Autodesk Inventor part; units mm, degrees
(part 3 of 6)
  line L915 (89.0625, 287.8731) -> (89.2677, 288.1729) construction
  line L916 (89.2677, 288.1729) -> (89.7412, 288.6466) construction
  line L917 (89.7412, 288.6466) -> (90.0412, 288.8519) construction
  line L918 (90.0412, 288.8519) -> (90.6984, 289.1241) construction
  line L919 (90.6984, 289.1241) -> (91.0556, 289.191) construction
  line L920 (91.0556, 289.191) -> (91.7253, 289.191) construction
  line L921 (91.7253, 289.191) -> (92.0826, 289.1241) construction
  line L922 (92.0826, 289.1241) -> (92.7397, 288.8518) construction
  line L923 (92.7397, 288.8518) -> (93.0397, 288.6465) construction
  line L924 (93.0397, 288.6465) -> (93.5132, 288.1729) construction
  line L925 (93.5132, 288.1729) -> (93.7184, 287.8731) construction
  line L926 (93.7184, 287.8731) -> (93.9905, 287.216) construction
  line L927 (93.9905, 287.216) -> (94.0574, 286.8589) construction
  line L928 (94.0574, 286.8589) -> (94.0574, 286.524) construction
  arc A169 (91.0729, 293.509) -> (84.7229, 287.159) centre (91.0729, 287.159) ccw
  arc A170 (98.6893, 291.9215) -> (97.1018, 293.509) centre (97.1018, 291.9215) ccw
  line L929 (97.1018, 293.509) -> (91.0729, 293.509)
  arc A171 (56.7829, 285.836) -> (57.2679, 280.4634) centre (86.7829, 285.836) ccw
  arc A172 (57.7529, 275.0908) -> (57.2679, 280.4634) centre (27.7529, 275.0908) ccw
  circle A173 centre (54.7529, 269.1865) radius 1.25
  arc A174 (61.7529, 277.269) -> (59.7529, 277.269) centre (60.7529, 277.269) ccw
  point P0 (0, 0)
  constraints: 242 point on circle, 232 end point, 175 centre point, 64 other
extrude "Extrusion1" add sketch "Sketch1" along normal blind 3.175
sketch "Sketch4" plane through (0, 3.175, 0) normal (0, 1, 0) x (1, 0, 0)
  line L0 (68.0533, -173.3296) -> (67.2896, -175.455) construction
  line L1 (67.2896, -175.455) -> (65.953, -179.1748) construction
  line L2 (65.953, -179.1748) -> (66.2895, -184.0091) construction
  line L3 (66.2895, -184.0091) -> (66.4824, -187.911) construction
  line L4 (66.4824, -187.911) -> (66.5623, -189.5259) construction
  line L5 (66.5623, -189.5259) -> (66.4659, -191.8029) construction
  line L6 (66.4659, -191.8029) -> (67.3465, -193.2223) construction
  line L7 (67.3465, -193.2223) -> (68.1874, -194.5775) construction
  line L8 (68.1874, -194.5775) -> (69.7981, -195.2031) construction
  line L9 (69.7981, -195.2031) -> (71.183, -194.3094) construction
  line L10 (71.183, -194.3094) -> (72.3101, -193.582) construction
  spline S0 degree 3 poles (71.4379, -191.0403) (71.4136, -190.7511) (71.3322, -190.3365) (71.3219, -190.1438) knots 8.458233 8.458233 8.458233 8.458233 9 9 9 9
  line L11 (71.3322, -190.3365) -> (71.3219, -190.1438) construction
  spline S1 degree 3 poles (71.3219, -190.1438) (71.2889, -189.5237) (71.258, -188.9035) (71.2265, -188.2833) knots 9 9 9 9 10 10 10 10
  line L12 (71.3219, -190.1438) -> (71.2889, -189.5237) construction
  line L13 (71.2889, -189.5237) -> (71.258, -188.9035) construction
  line L14 (71.258, -188.9035) -> (71.2265, -188.2833) construction
  line L15 (71.2265, -188.2833) -> (71.1692, -187.1534) construction
  line L16 (54.8134, -176.6589) -> (58.7542, -172.8132) construction
  line L17 (58.7542, -172.8132) -> (63.5056, -170.1212) construction
  line L18 (63.5056, -170.1212) -> (69.0045, -169.3212) construction
  line L19 (69.0045, -169.3212) -> (70.5265, -169.0997) construction
  line L20 (70.5265, -169.0997) -> (74.7787, -168.4041) construction
  line L21 (74.7787, -168.4041) -> (75.871, -170.0274) construction
  line L22 (75.871, -170.0274) -> (76.7396, -171.3185) construction
  line L23 (70.8964, -175.7745) -> (70.6915, -175.9124) construction
  line L24 (70.6915, -175.9124) -> (68.7543, -177.2158) construction
  line L25 (68.7543, -177.2158) -> (66.0254, -178.5253) construction
  line L26 (66.0254, -178.5253) -> (66.5069, -181.34) construction
  line L27 (66.5069, -181.34) -> (67.038, -184.4454) construction
  line L28 (67.038, -184.4454) -> (70.5258, -184.7447) construction
  line L29 (70.5258, -184.7447) -> (73.0271, -185.2813) construction
  line L30 (73.0271, -185.2813) -> (74.5567, -185.6094) construction
  line L31 (74.5567, -185.6094) -> (76.0864, -185.9375) construction
  line L32 (76.0864, -185.9375) -> (77.616, -186.2656) construction
  line L33 (77.616, -186.2656) -> (78.6507, -186.4876) construction
  line L34 (78.6507, -186.4876) -> (80.7148, -186.605) construction
  line L35 (80.7148, -186.605) -> (81.3787, -187.5477) construction
  line L36 (81.3787, -187.5477) -> (82.8031, -189.5702) construction
  line L37 (82.8031, -189.5702) -> (78.7693, -192.6215) construction
  line L38 (78.7693, -192.6215) -> (77.5691, -193.7926) construction
  line L39 (77.5691, -193.7926) -> (75.0315, -196.2689) construction
  line L40 (75.0315, -196.2689) -> (72.0888, -198.6438) construction
  line L41 (72.0888, -198.6438) -> (69.9041, -201.4382) construction
  line L42 (69.9041, -201.4382) -> (67.9877, -203.8893) construction
  line L43 (67.9877, -203.8893) -> (67.3791, -207.1454) construction
  line L44 (67.3791, -207.1454) -> (70.2519, -209.1046) construction
  line L45 (70.2519, -209.1046) -> (72.2021, -210.4346) construction
  line L46 (72.2021, -210.4346) -> (74.2923, -207.8924) construction
  line L47 (74.2923, -207.8924) -> (73.3096, -206.0468) construction
  line L48 (73.3096, -206.0468) -> (72.9443, -205.3608) construction
  line L49 (72.9443, -205.3608) -> (74.6423, -203.8692) construction
  line L50 (74.6423, -203.8692) -> (75.0347, -203.4711) construction
  line L51 (75.0347, -203.4711) -> (76.3526, -202.1342) construction
  line L52 (76.3526, -202.1342) -> (77.6846, -200.8109) construction
  line L53 (77.6846, -200.8109) -> (79.0094, -199.4809) construction
  line L54 (79.0094, -199.4809) -> (81.2117, -197.27) construction
  line L55 (81.2117, -197.27) -> (83.979, -195.0838) construction
  line L56 (83.979, -195.0838) -> (85.5163, -192.3208) construction
  line L57 (85.5163, -192.3208) -> (86.9983, -189.6573) construction
  line L58 (86.9983, -189.6573) -> (87.0793, -186.0473) construction
  line L59 (87.0793, -186.0473) -> (84.7384, -183.8306) construction
  line L60 (84.7384, -183.8306) -> (82.5192, -181.7291) construction
  line L61 (82.5192, -181.7291) -> (78.9491, -181.4958) construction
  line L62 (78.9491, -181.4958) -> (76.1047, -180.8984) construction
  line L63 (76.1047, -180.8984) -> (75.2801, -180.7252) construction
  line L64 (75.2801, -180.7252) -> (74.4555, -180.552) construction
  line L65 (74.4555, -180.552) -> (73.6309, -180.3788) construction
  line L66 (73.6309, -180.3788) -> (73.4532, -180.3415) construction
  spline S2 degree 3 poles (72.7888, -180.137) (73.3091, -179.7654) (73.8195, -179.3794) (74.3176, -178.9789) (76.5193, -177.2088) (79.468, -174.7132) (80.2974, -171.9013) (82.2261, -165.3626) (73.6813, -164.3195) (69.3125, -164.8443) (62.769, -165.6304) (56.2883, -168.7774) (52.0514, -173.8969) (50.4747, -175.8021) (52.9801, -178.448) (54.8134, -176.6589) knots 21.261625 21.261625 21.261625 21.261625 22 22 22 23 23 23 24 24 24 25 25 25 26 26 26 26
  line L67 (73.8195, -179.3794) -> (74.3176, -178.9789) construction
  line L68 (74.3176, -178.9789) -> (76.5193, -177.2088) construction
  line L69 (76.5193, -177.2088) -> (79.468, -174.7132) construction
  line L70 (79.468, -174.7132) -> (80.2974, -171.9013) construction
  line L71 (80.2974, -171.9013) -> (82.2261, -165.3626) construction
  line L72 (82.2261, -165.3626) -> (73.6813, -164.3195) construction
  line L73 (73.6813, -164.3195) -> (69.3125, -164.8443) construction
  line L74 (69.3125, -164.8443) -> (62.769, -165.6304) construction
  line L75 (62.769, -165.6304) -> (56.2883, -168.7774) construction
  line L76 (56.2883, -168.7774) -> (52.0514, -173.8969) construction
  line L77 (52.0514, -173.8969) -> (50.4747, -175.8021) construction
  line L78 (50.4747, -175.8021) -> (52.9801, -178.448) construction
  line L79 (52.9801, -178.448) -> (54.8134, -176.6589) construction
  line L80 (82.6309, -166.8487) -> (78.6495, -169.856) construction
  line L81 (78.6495, -169.856) -> (78.7473, -175.7342) construction
  line L82 (78.7473, -175.7342) -> (82.8138, -178.6713) construction
  line L83 (82.8138, -178.6713) -> (85.2708, -180.4459) construction
  line L84 (96.4523, -176.1121) -> (96.5051, -176.048) construction
  line L85 (96.5051, -176.048) -> (98.1056, -174.1068) construction
  line L86 (98.1056, -174.1068) -> (99.723, -171.3331) construction
  line L87 (99.723, -171.3331) -> (98.0656, -168.9339) construction
  line L88 (98.0656, -168.9339) -> (96.4673, -166.6204) construction
  line L89 (96.4673, -166.6204) -> (93.1935, -166.91) construction
  line L90 (93.1935, -166.91) -> (91.8605, -169.3049) construction
  line L91 (91.8605, -169.3049) -> (91.0125, -170.8285) construction
  line L92 (90.509, -185.6944) -> (90.2633, -188.6117) construction
  line L93 (90.2633, -188.6117) -> (89.9424, -192.421) construction
  line L94 (89.9424, -192.421) -> (89.5263, -196.2245) construction
  line L95 (89.5263, -196.2245) -> (88.9864, -200.0092) construction
  line L96 (88.9864, -200.0092) -> (88.4414, -203.8299) construction
  line L97 (88.4414, -203.8299) -> (87.5894, -207.7568) construction
  line L98 (87.5894, -207.7568) -> (87.62, -211.6254) construction
  line L99 (87.62, -211.6254) -> (87.6402, -214.1845) construction
  line L100 (87.6402, -214.1845) -> (90.9164, -214.2859) construction
  line L101 (90.9164, -214.2859) -> (91.7855, -212.1891) construction
  line L102 (91.7855, -212.1891) -> (93.8827, -207.1293) construction
  line L103 (93.8827, -207.1293) -> (94.3063, -201.2098) construction
  line L104 (94.3063, -201.2098) -> (94.9587, -195.8163) construction
  line L105 (94.9587, -195.8163) -> (95.6151, -190.39) construction
  line L106 (95.6151, -190.39) -> (96.0487, -184.9444) construction
  line L107 (96.0487, -184.9444) -> (96.2472, -179.4821) construction
  line L108 (96.2472, -179.4821) -> (96.2865, -178.4016) construction
  spline S3 degree 3 poles (90.9094, -174.8252) (90.69, -174.9606) (90.4623, -175.0836) (90.2255, -175.1921) (88.4887, -175.9878) (86.0785, -175.8652) (84.7267, -174.3834) (83.5291, -173.0705) (83.7173, -171.0568) (84.9977, -169.9161) (86.6252, -168.4662) (84.4158, -165.5005) (82.6309, -166.8487) knots 16.74527 16.74527 16.74527 16.74527 17 17 17 18 18 18 19 19 19 20 20 20 20
  line L109 (90.4623, -175.0836) -> (90.2255, -175.1921) construction
  line L110 (90.2255, -175.1921) -> (88.4887, -175.9878) construction
  line L111 (88.4887, -175.9878) -> (86.0785, -175.8652) construction
  line L112 (86.0785, -175.8652) -> (84.7267, -174.3834) construction
  line L113 (84.7267, -174.3834) -> (83.5291, -173.0705) construction
  line L114 (83.5291, -173.0705) -> (83.7173, -171.0568) construction
  line L115 (83.7173, -171.0568) -> (84.9977, -169.9161) construction
  line L116 (84.9977, -169.9161) -> (86.6252, -168.4662) construction
  line L117 (86.6252, -168.4662) -> (84.4158, -165.5005) construction
  line L118 (84.4158, -165.5005) -> (82.6309, -166.8487) construction
  line L119 (90.69, -174.9606) -> (90.4623, -175.0836) construction
  line L120 (90.9094, -174.8252) -> (90.69, -174.9606) construction
  spline S4 degree 3 poles (96.3446, -176.2385) (96.3988, -176.1756) (96.4523, -176.1121) (96.5051, -176.048) (98.1056, -174.1068) (99.723, -171.3331) (98.0656, -168.9339) (96.4673, -166.6204) (93.1935, -166.91) (91.8605, -169.3049) (91.0125, -170.8285) (90.8978, -172.8553) (90.9094, -174.8252) knots 1.983848 1.983848 1.983848 1.983848 2 2 2 3 3 3 4 4 4 4.613609 4.613609 4.613609 4.613609
  line L121 (91.0125, -170.8285) -> (90.8978, -172.8553) construction
  line L122 (90.8978, -172.8553) -> (90.9094, -174.8252) construction
  line L123 (90.7165, -182.7739) -> (90.509, -185.6944) construction
  line L124 (90.8611, -179.8499) -> (90.7165, -182.7739) construction
  spline S5 degree 3 poles (82.6309, -166.8487) (78.6495, -169.856) (78.7473, -175.7342) (82.8138, -178.6713) (85.2708, -180.4459) (88.1892, -180.6709) (90.8611, -179.8499) knots 0 0 0 0 1 1 1 1.551759 1.551759 1.551759 1.551759
  line L125 (85.2708, -180.4459) -> (88.1892, -180.6709) construction
  line L126 (88.1892, -180.6709) -> (90.8611, -179.8499) construction
  line L127 (96.3988, -176.1756) -> (96.4523, -176.1121) construction
  line L128 (96.3446, -176.2385) -> (96.3988, -176.1756) construction
  spline S6 degree 3 poles (90.8611, -179.8499) (90.7165, -182.7739) (90.509, -185.6944) (90.2633, -188.6117) (89.9424, -192.421) (89.5263, -196.2245) (88.9864, -200.0092) (88.4414, -203.8299) (87.5894, -207.7568) (87.62, -211.6254) (87.6402, -214.1845) (90.9164, -214.2859) (91.7855, -212.1891) (93.8827, -207.1293) (94.3063, -201.2098) (94.9587, -195.8163) (95.6151, -190.39) (96.0487, -184.9444) (96.2472, -179.4821) (96.2865, -178.4016) (96.3238, -177.32) (96.3446, -176.2385) knots 5.14687 5.14687 5.14687 5.14687 6 6 6 7 7 7 8 8 8 9 9 9 10 10 10 11 11 11 11.773986 11.773986 11.773986 11.773986
  line L129 (96.2865, -178.4016) -> (96.3238, -177.32) construction
  line L130 (96.3238, -177.32) -> (96.3446, -176.2385) construction
  spline S7 degree 3 poles (54.8134, -176.6589) (58.7542, -172.8132) (63.5056, -170.1212) (69.0045, -169.3212) (70.5265, -169.0997) (74.7787, -168.4041) (75.871, -170.0274) (76.7396, -171.3185) (72.8595, -174.3629) (71.2168, -175.5448) knots 0 0 0 0 1 1 1 2 2 2 2.88117 2.88117 2.88117 2.88117
  line L131 (76.7396, -171.3185) -> (72.8595, -174.3629) construction
  line L132 (72.8595, -174.3629) -> (71.2168, -175.5448) construction
  line L133 (70.9953, -175.7041) -> (70.8964, -175.7745) construction
  line L134 (71.2168, -175.5448) -> (70.9953, -175.7041) construction
  line L135 (73.3091, -179.7654) -> (73.8195, -179.3794) construction
  line L136 (72.7888, -180.137) -> (73.3091, -179.7654) construction
  spline S8 degree 3 poles (71.2168, -175.5448) (70.9953, -175.7041) (70.8964, -175.7745) (70.6915, -175.9124) (68.7543, -177.2158) (66.0254, -178.5253) (66.5069, -181.34) (67.038, -184.4454) (70.5258, -184.7447) (73.0271, -185.2813) (74.5567, -185.6094) (76.0864, -185.9375) (77.616, -186.2656) (78.6507, -186.4876) (80.7148, -186.605) (81.3787, -187.5477) (82.8031, -189.5702) (78.7693, -192.6215) (77.5691, -193.7926) (75.0315, -196.2689) (72.0888, -198.6438) (69.9041, -201.4382) (67.9877, -203.8893) (67.3791, -207.1454) (70.2519, -209.1046) (72.2021, -210.4346) (74.2923, -207.8924) (73.3096, -206.0468) (72.9443, -205.3608) (74.6423, -203.8692) (75.0347, -203.4711) (76.3526, -202.1342) (77.6846, -200.8109) (79.0094, -199.4809) (81.2117, -197.27) (83.979, -195.0838) (85.5163, -192.3208) (86.9983, -189.6573) (87.0793, -186.0473) (84.7384, -183.8306) (82.5192, -181.7291) (78.9491, -181.4958) (76.1047, -180.8984) (75.2801, -180.7252) (74.4555, -180.552) (73.6309, -180.3788) (73.4532, -180.3415) (73.1367, -180.241) (72.7888, -180.137) knots 2.88117 2.88117 2.88117 2.88117 3 3 3 4 4 4 5 5 5 6 6 6 7 7 7 8 8 8 9 9 9 10 10 10 11 11 11 12 12 12 13 13 13 14 14 14 15 15 15 16 16 16 17 17 17 17.368094 17.368094 17.368094 17.368094
  line L137 (73.4532, -180.3415) -> (73.1367, -180.241) construction
  line L138 (73.1367, -180.241) -> (72.7888, -180.137) construction
  spline S9 degree 3 poles (71.2265, -188.2833) (71.1692, -187.1534) (71.1235, -186.0243) (71.1084, -184.8935) knots 10 10 10 10 10.82684 10.82684 10.82684 10.82684
  line L139 (71.1692, -187.1534) -> (71.1235, -186.0243) construction
  line L140 (71.1235, -186.0243) -> (71.1084, -184.8935) construction
  line L141 (70.7832, -173.7477) -> (68.0533, -173.3296) construction
  line L142 (71.2168, -175.5448) -> (70.7832, -173.7477) construction
  spline S10 degree 3 poles (71.2168, -175.5448) (70.7832, -173.7477) (68.0533, -173.3296) (67.2896, -175.455) (65.953, -179.1748) (66.2895, -184.0091) (66.4824, -187.911) (66.5623, -189.5259) (66.4659, -191.8029) (67.3465, -193.2223) (68.1874, -194.5775) (69.7981, -195.2031) (71.183, -194.3094) (72.3101, -193.582) (72.3478, -191.8168) (71.4379, -191.0403) knots 1.141449 1.141449 1.141449 1.141449 2 2 2 3 3 3 4 4 4 5 5 5 5.747549 5.747549 5.747549 5.747549
  line L143 (72.3101, -193.582) -> (72.3478, -191.8168) construction
  line L144 (72.3478, -191.8168) -> (71.4379, -191.0403) construction
  line L145 (71.4136, -190.7511) -> (71.3322, -190.3365) construction
  line L146 (71.4379, -191.0403) -> (71.4136, -190.7511) construction
  point P0 (0, 0)
  point P1 (71.2746, -176.0007)
  constraints: 30 other
extrude "Extrusion3" add sketch "Sketch4" against normal up to surface (3.175 mm away)
sketch "Sketch5" plane through (0, 3.175, 0) normal (0, 1, 0) x (1, 0, 0)
  circle A0 centre (94.9575, -171.3179) radius 1.9844
  point P0 (0, 0)
  dimension "d9" = 3.9688
  constraints: 1 centre point
  measures "d9" diameter of A0
extrude "Extrusion4" cut sketch "Sketch5" against normal through all
sketch "Sketch6" plane through (0, 3.175, 0) normal (0, 1, 0) x (1, 0, 0)
  line L0 (-91.0753, -197.2079) -> (-91.3616, -198.0049) construction
  line L1 (-91.3616, -198.0049) -> (-91.8629, -199.3998) construction
  line L2 (-91.8629, -199.3998) -> (-91.7367, -201.2127) construction
  line L3 (-91.7367, -201.2127) -> (-91.6643, -202.6759) construction
  line L4 (-91.6643, -202.6759) -> (-91.6344, -203.2815) construction
  line L5 (-91.6344, -203.2815) -> (-91.6705, -204.1354) construction
  line L6 (-91.6705, -204.1354) -> (-91.3403, -204.6676) construction
  line L7 (-91.3403, -204.6676) -> (-91.025, -205.1759) construction
  line L8 (-91.025, -205.1759) -> (-90.4209, -205.4105) construction
  line L9 (-90.4209, -205.4105) -> (-89.9016, -205.0753) construction
  line L10 (-89.9016, -205.0753) -> (-89.479, -204.8025) construction
  spline S0 degree 3 poles (-89.806, -203.8494) (-89.8151, -203.7409) (-89.8457, -203.5855) (-89.8495, -203.5132) knots 8.458233 8.458233 8.458233 8.458233 9 9 9 9
  line L11 (-89.8457, -203.5855) -> (-89.8495, -203.5132) construction
  spline S1 degree 3 poles (-89.8495, -203.5132) (-89.8619, -203.2807) (-89.8735, -203.0481) (-89.8853, -202.8155) knots 9 9 9 9 10 10 10 10
  line L12 (-89.8495, -203.5132) -> (-89.8619, -203.2807) construction
  line L13 (-89.8619, -203.2807) -> (-89.8735, -203.0481) construction
  line L14 (-89.8735, -203.0481) -> (-89.8853, -202.8155) construction
  line L15 (-89.8853, -202.8155) -> (-89.9068, -202.3918) construction
  line L16 (-96.0402, -198.4564) -> (-94.5624, -197.0142) construction
  line L17 (-94.5624, -197.0142) -> (-92.7806, -196.0047) construction
  line L18 (-92.7806, -196.0047) -> (-90.7186, -195.7047) construction
  line L19 (-90.7186, -195.7047) -> (-90.1478, -195.6217) construction
  line L20 (-90.1478, -195.6217) -> (-88.5532, -195.3608) construction
  line L21 (-88.5532, -195.3608) -> (-88.1436, -195.9696) construction
  line L22 (-88.1436, -195.9696) -> (-87.8179, -196.4537) construction
  line L23 (-90.0091, -198.1247) -> (-90.0859, -198.1764) construction
  line L24 (-90.0859, -198.1764) -> (-90.8124, -198.6652) construction
  line L25 (-90.8124, -198.6652) -> (-91.8357, -199.1563) construction
  line L26 (-91.8357, -199.1563) -> (-91.6552, -200.2118) construction
  line L27 (-91.6552, -200.2118) -> (-91.456, -201.3763) construction
  line L28 (-91.456, -201.3763) -> (-90.1481, -201.4886) construction
  line L29 (-90.1481, -201.4886) -> (-89.2101, -201.6898) construction
  line L30 (-89.2101, -201.6898) -> (-88.6365, -201.8128) construction
  line L31 (-88.6365, -201.8128) -> (-88.0628, -201.9358) construction
  line L32 (-88.0628, -201.9358) -> (-87.4892, -202.0589) construction
  line L33 (-87.4892, -202.0589) -> (-87.1012, -202.1421) construction
  line L34 (-87.1012, -202.1421) -> (-86.3272, -202.1861) construction
  line L35 (-86.3272, -202.1861) -> (-86.0782, -202.5397) construction
  line L36 (-86.0782, -202.5397) -> (-85.5441, -203.2981) construction
  line L37 (-85.5441, -203.2981) -> (-87.0568, -204.4423) construction
  line L38 (-87.0568, -204.4423) -> (-87.5068, -204.8815) construction
  line L39 (-87.5068, -204.8815) -> (-88.4584, -205.8101) construction
  line L40 (-88.4584, -205.8101) -> (-89.5619, -206.7007) construction
  line L41 (-89.5619, -206.7007) -> (-90.3812, -207.7486) construction
  line L42 (-90.3812, -207.7486) -> (-91.0998, -208.6678) construction
  line L43 (-91.0998, -208.6678) -> (-91.3281, -209.8888) construction
  line L44 (-91.3281, -209.8888) -> (-90.2508, -210.6235) construction
  line L45 (-90.2508, -210.6235) -> (-89.5194, -211.1222) construction
  line L46 (-89.5194, -211.1222) -> (-88.7356, -210.1689) construction
  line L47 (-88.7356, -210.1689) -> (-89.1041, -209.4768) construction
  line L48 (-89.1041, -209.4768) -> (-89.2411, -209.2196) construction
  line L49 (-89.2411, -209.2196) -> (-88.6044, -208.6602) construction
  line L50 (-88.6044, -208.6602) -> (-88.4572, -208.5109) construction
  line L51 (-88.4572, -208.5109) -> (-87.963, -208.0096) construction
  line L52 (-87.963, -208.0096) -> (-87.4635, -207.5134) construction
  line L53 (-87.4635, -207.5134) -> (-86.9667, -207.0146) construction
  line L54 (-86.9667, -207.0146) -> (-86.1408, -206.1855) construction
  line L55 (-86.1408, -206.1855) -> (-85.1031, -205.3657) construction
  line L56 (-85.1031, -205.3657) -> (-84.5266, -204.3296) construction
  line L57 (-84.5266, -204.3296) -> (-83.9709, -203.3308) construction
  line L58 (-83.9709, -203.3308) -> (-83.9405, -201.977) construction
  line L59 (-83.9405, -201.977) -> (-84.8183, -201.1457) construction
  line L60 (-84.8183, -201.1457) -> (-85.6505, -200.3577) construction
  line L61 (-85.6505, -200.3577) -> (-86.9893, -200.2702) construction
  line L62 (-86.9893, -200.2702) -> (-88.056, -200.0462) construction
  line L63 (-88.056, -200.0462) -> (-88.3652, -199.9812) construction
  line L64 (-88.3652, -199.9812) -> (-88.6744, -199.9163) construction
  line L65 (-88.6744, -199.9163) -> (-88.9837, -199.8513) construction
  line L66 (-88.9837, -199.8513) -> (-89.0503, -199.8373) construction
  spline S2 degree 3 poles (-89.2994, -199.7606) (-89.1043, -199.6213) (-88.9129, -199.4765) (-88.7261, -199.3264) (-87.9005, -198.6626) (-86.7947, -197.7267) (-86.4837, -196.6723) (-85.7604, -194.2202) (-88.9647, -193.8291) (-90.603, -194.0259) (-93.0568, -194.3207) (-95.4871, -195.5008) (-97.076, -197.4206) (-97.6672, -198.1351) (-96.7277, -199.1273) (-96.0402, -198.4564) knots 21.261625 21.261625 21.261625 21.261625 22 22 22 23 23 23 24 24 24 25 25 25 26 26 26 26
  line L67 (-88.9129, -199.4765) -> (-88.7261, -199.3264) construction
  line L68 (-88.7261, -199.3264) -> (-87.9005, -198.6626) construction
  line L69 (-87.9005, -198.6626) -> (-86.7947, -197.7267) construction
  line L70 (-86.7947, -197.7267) -> (-86.4837, -196.6723) construction
  line L71 (-86.4837, -196.6723) -> (-85.7604, -194.2202) construction
  line L72 (-85.7604, -194.2202) -> (-88.9647, -193.8291) construction
  line L73 (-88.9647, -193.8291) -> (-90.603, -194.0259) construction
  line L74 (-90.603, -194.0259) -> (-93.0568, -194.3207) construction
  line L75 (-93.0568, -194.3207) -> (-95.4871, -195.5008) construction
  line L76 (-95.4871, -195.5008) -> (-97.076, -197.4206) construction
  line L77 (-97.076, -197.4206) -> (-97.6672, -198.1351) construction
  line L78 (-97.6672, -198.1351) -> (-96.7277, -199.1273) construction
  line L79 (-96.7277, -199.1273) -> (-96.0402, -198.4564) construction
  line L80 (-85.6086, -194.7775) -> (-87.1017, -195.9053) construction
  line L81 (-87.1017, -195.9053) -> (-87.065, -198.1096) construction
  line L82 (-87.065, -198.1096) -> (-85.54, -199.211) construction
  line L83 (-85.54, -199.211) -> (-84.6187, -199.8765) construction
  line L84 (-80.4256, -198.2513) -> (-80.4058, -198.2273) construction
  line L85 (-80.4058, -198.2273) -> (-79.8056, -197.4993) construction
  line L86 (-79.8056, -197.4993) -> (-79.1991, -196.4592) construction
  line L87 (-79.1991, -196.4592) -> (-79.8206, -195.5595) construction
  line L88 (-79.8206, -195.5595) -> (-80.42, -194.6919) construction
  line L89 (-80.42, -194.6919) -> (-81.6477, -194.8005) construction
  line L90 (-81.6477, -194.8005) -> (-82.1475, -195.6986) construction
  line L91 (-82.1475, -195.6986) -> (-82.4655, -196.27) construction
  line L92 (-82.6543, -201.8447) -> (-82.7465, -202.9386) construction
  line L93 (-82.7465, -202.9386) -> (-82.8668, -204.3672) construction
  line L94 (-82.8668, -204.3672) -> (-83.0229, -205.7935) construction
  line L95 (-83.0229, -205.7935) -> (-83.2253, -207.2127) construction
  line L96 (-83.2253, -207.2127) -> (-83.4297, -208.6455) construction
  line L97 (-83.4297, -208.6455) -> (-83.7492, -210.1181) construction
  line L98 (-83.7492, -210.1181) -> (-83.7377, -211.5688) construction
  line L99 (-83.7377, -211.5688) -> (-83.7302, -212.5285) construction
  line L100 (-83.7302, -212.5285) -> (-82.5016, -212.5665) construction
  line L101 (-82.5016, -212.5665) -> (-82.1757, -211.7802) construction
  line L102 (-82.1757, -211.7802) -> (-81.3892, -209.8828) construction
  line L103 (-81.3892, -209.8828) -> (-81.2304, -207.6629) construction
  line L104 (-81.2304, -207.6629) -> (-80.9857, -205.6404) construction
  line L105 (-80.9857, -205.6404) -> (-80.7396, -203.6055) construction
  line L106 (-80.7396, -203.6055) -> (-80.577, -201.5634) construction
  line L107 (-80.577, -201.5634) -> (-80.5025, -199.5151) construction
  line L108 (-80.5025, -199.5151) -> (-80.4878, -199.1099) construction
  spline S3 degree 3 poles (-82.5042, -197.7687) (-82.5865, -197.8195) (-82.6719, -197.8656) (-82.7607, -197.9063) (-83.412, -198.2047) (-84.3158, -198.1587) (-84.8227, -197.603) (-85.2718, -197.1107) (-85.2012, -196.3556) (-84.7211, -195.9278) (-84.1108, -195.3841) (-84.9393, -194.272) (-85.6086, -194.7775) knots 16.74527 16.74527 16.74527 16.74527 17 17 17 18 18 18 19 19 19 20 20 20 20
  line L109 (-82.6719, -197.8656) -> (-82.7607, -197.9063) construction
  line L110 (-82.7607, -197.9063) -> (-83.412, -198.2047) construction
  line L111 (-83.412, -198.2047) -> (-84.3158, -198.1587) construction
  line L112 (-84.3158, -198.1587) -> (-84.8227, -197.603) construction
  line L113 (-84.8227, -197.603) -> (-85.2718, -197.1107) construction
  line L114 (-85.2718, -197.1107) -> (-85.2012, -196.3556) construction
  line L115 (-85.2012, -196.3556) -> (-84.7211, -195.9278) construction
  line L116 (-84.7211, -195.9278) -> (-84.1108, -195.3841) construction
  line L117 (-84.1108, -195.3841) -> (-84.9393, -194.272) construction
  line L118 (-84.9393, -194.272) -> (-85.6086, -194.7775) construction
  line L119 (-82.5865, -197.8195) -> (-82.6719, -197.8656) construction
  line L120 (-82.5042, -197.7687) -> (-82.5865, -197.8195) construction
  spline S4 degree 3 poles (-80.466, -198.2987) (-80.4457, -198.2751) (-80.4256, -198.2513) (-80.4058, -198.2273) (-79.8056, -197.4993) (-79.1991, -196.4592) (-79.8206, -195.5595) (-80.42, -194.6919) (-81.6477, -194.8005) (-82.1475, -195.6986) (-82.4655, -196.27) (-82.5086, -197.03) (-82.5042, -197.7687) knots 1.983848 1.983848 1.983848 1.983848 2 2 2 3 3 3 4 4 4 4.613609 4.613609 4.613609 4.613609
  line L121 (-82.4655, -196.27) -> (-82.5086, -197.03) construction
  line L122 (-82.5086, -197.03) -> (-82.5042, -197.7687) construction
  line L123 (-82.5765, -200.7495) -> (-82.6543, -201.8447) construction
  line L124 (-82.5223, -199.653) -> (-82.5765, -200.7495) construction
  spline S5 degree 3 poles (-85.6086, -194.7775) (-87.1017, -195.9053) (-87.065, -198.1096) (-85.54, -199.211) (-84.6187, -199.8765) (-83.5243, -199.9609) (-82.5223, -199.653) knots 0 0 0 0 1 1 1 1.551759 1.551759 1.551759 1.551759
  line L125 (-84.6187, -199.8765) -> (-83.5243, -199.9609) construction
  line L126 (-83.5243, -199.9609) -> (-82.5223, -199.653) construction
  line L127 (-80.4457, -198.2751) -> (-80.4256, -198.2513) construction
  line L128 (-80.466, -198.2987) -> (-80.4457, -198.2751) construction
  spline S6 degree 3 poles (-82.5223, -199.653) (-82.5765, -200.7495) (-82.6543, -201.8447) (-82.7465, -202.9386) (-82.8668, -204.3672) (-83.0229, -205.7935) (-83.2253, -207.2127) (-83.4297, -208.6455) (-83.7492, -210.1181) (-83.7377, -211.5688) (-83.7302, -212.5285) (-82.5016, -212.5665) (-82.1757, -211.7802) (-81.3892, -209.8828) (-81.2304, -207.6629) (-80.9857, -205.6404) (-80.7396, -203.6055) (-80.577, -201.5634) (-80.5025, -199.5151) (-80.4878, -199.1099) (-80.4738, -198.7043) (-80.466, -198.2987) knots 5.14687 5.14687 5.14687 5.14687 6 6 6 7 7 7 8 8 8 9 9 9 10 10 10 11 11 11 11.773986 11.773986 11.773986 11.773986
  line L129 (-80.4878, -199.1099) -> (-80.4738, -198.7043) construction
  line L130 (-80.4738, -198.7043) -> (-80.466, -198.2987) construction
  spline S7 degree 3 poles (-96.0402, -198.4564) (-94.5624, -197.0142) (-92.7806, -196.0047) (-90.7186, -195.7047) (-90.1478, -195.6217) (-88.5532, -195.3608) (-88.1436, -195.9696) (-87.8179, -196.4537) (-89.2729, -197.5954) (-89.8889, -198.0386) knots 0 0 0 0 1 1 1 2 2 2 2.88117 2.88117 2.88117 2.88117
  line L131 (-87.8179, -196.4537) -> (-89.2729, -197.5954) construction
  line L132 (-89.2729, -197.5954) -> (-89.8889, -198.0386) construction
  line L133 (-89.972, -198.0983) -> (-90.0091, -198.1247) construction
  line L134 (-89.8889, -198.0386) -> (-89.972, -198.0983) construction
  line L135 (-89.1043, -199.6213) -> (-88.9129, -199.4765) construction
  line L136 (-89.2994, -199.7606) -> (-89.1043, -199.6213) construction
  spline S8 degree 3 poles (-89.8889, -198.0386) (-89.972, -198.0983) (-90.0091, -198.1247) (-90.0859, -198.1764) (-90.8124, -198.6652) (-91.8357, -199.1563) (-91.6552, -200.2118) (-91.456, -201.3763) (-90.1481, -201.4886) (-89.2101, -201.6898) (-88.6365, -201.8128) (-88.0628, -201.9358) (-87.4892, -202.0589) (-87.1012, -202.1421) (-86.3272, -202.1861) (-86.0782, -202.5397) (-85.5441, -203.2981) (-87.0568, -204.4423) (-87.5068, -204.8815) (-88.4584, -205.8101) (-89.5619, -206.7007) (-90.3812, -207.7486) (-91.0998, -208.6678) (-91.3281, -209.8888) (-90.2508, -210.6235) (-89.5194, -211.1222) (-88.7356, -210.1689) (-89.1041, -209.4768) (-89.2411, -209.2196) (-88.6044, -208.6602) (-88.4572, -208.5109) (-87.963, -208.0096) (-87.4635, -207.5134) (-86.9667, -207.0146) (-86.1408, -206.1855) (-85.1031, -205.3657) (-84.5266, -204.3296) (-83.9709, -203.3308) (-83.9405, -201.977) (-84.8183, -201.1457) (-85.6505, -200.3577) (-86.9893, -200.2702) (-88.056, -200.0462) (-88.3652, -199.9812) (-88.6744, -199.9163) (-88.9837, -199.8513) (-89.0503, -199.8373) (-89.169, -199.7996) (-89.2994, -199.7606) knots 2.88117 2.88117 2.88117 2.88117 3 3 3 4 4 4 5 5 5 6 6 6 7 7 7 8 8 8 9 9 9 10 10 10 11 11 11 12 12 12 13 13 13 14 14 14 15 15 15 16 16 16 17 17 17 17.368094 17.368094 17.368094 17.368094
  line L137 (-89.0503, -199.8373) -> (-89.169, -199.7996) construction
  line L138 (-89.169, -199.7996) -> (-89.2994, -199.7606) construction
  spline S9 degree 3 poles (-89.8853, -202.8155) (-89.9068, -202.3918) (-89.9239, -201.9684) (-89.9296, -201.5443) knots 10 10 10 10 10.82684 10.82684 10.82684 10.82684
  line L139 (-89.9068, -202.3918) -> (-89.9239, -201.9684) construction
  line L140 (-89.9239, -201.9684) -> (-89.9296, -201.5443) construction
  line L141 (-90.0515, -197.3647) -> (-91.0753, -197.2079) construction
  line L142 (-89.8889, -198.0386) -> (-90.0515, -197.3647) construction
  spline S10 degree 3 poles (-89.8889, -198.0386) (-90.0515, -197.3647) (-91.0753, -197.2079) (-91.3616, -198.0049) (-91.8629, -199.3998) (-91.7367, -201.2127) (-91.6643, -202.6759) (-91.6344, -203.2815) (-91.6705, -204.1354) (-91.3403, -204.6676) (-91.025, -205.1759) (-90.4209, -205.4105) (-89.9016, -205.0753) (-89.479, -204.8025) (-89.4648, -204.1406) (-89.806, -203.8494) knots 1.141449 1.141449 1.141449 1.141449 2 2 2 3 3 3 4 4 4 5 5 5 5.747549 5.747549 5.747549 5.747549
  line L143 (-89.479, -204.8025) -> (-89.4648, -204.1406) construction
  line L144 (-89.4648, -204.1406) -> (-89.806, -203.8494) construction
  line L145 (-89.8151, -203.7409) -> (-89.8457, -203.5855) construction
  line L146 (-89.806, -203.8494) -> (-89.8151, -203.7409) construction
  circle A0 centre (-80.9398, -196.4592) radius 0.6286
  line L147 (-44.4004, -216.039) -> (-97.1018, -216.039) projected
  line L148 (-42.8129, -292.5565) -> (-42.8129, -217.6265) projected
  line L149 (-71.1319, -207.3346) -> (-70.5279, -207.5692) construction
  spline S11 degree 3 poles (-69.9958, -200.1973) (-70.1585, -199.5234) (-71.1822, -199.3666) (-71.4686, -200.1636) (-71.9698, -201.5585) (-71.8436, -203.3714) (-71.7713, -204.8346) (-71.7413, -205.4402) (-71.7775, -206.2941) (-71.4472, -206.8263) (-71.1319, -207.3346) (-70.5279, -207.5692) (-70.0086, -207.234) (-69.5859, -206.9613) (-69.5717, -206.2993) (-69.913, -206.0081) knots 1.141449 1.141449 1.141449 1.141449 2 2 2 3 3 3 4 4 4 5 5 5 5.747549 5.747549 5.747549 5.747549
  line L150 (-69.9958, -200.1973) -> (-70.1585, -199.5234) construction
  line L151 (-70.1585, -199.5234) -> (-71.1822, -199.3666) construction
  line L152 (-71.1822, -199.3666) -> (-71.4686, -200.1636) construction
  line L153 (-71.4686, -200.1636) -> (-71.9698, -201.5585) construction
  line L154 (-71.9698, -201.5585) -> (-71.8436, -203.3714) construction
  line L155 (-71.8436, -203.3714) -> (-71.7713, -204.8346) construction
  line L156 (-71.7713, -204.8346) -> (-71.7413, -205.4402) construction
  line L157 (-71.7413, -205.4402) -> (-71.7775, -206.2941) construction
  line L158 (-71.7775, -206.2941) -> (-71.4472, -206.8263) construction
  line L159 (-71.4472, -206.8263) -> (-71.1319, -207.3346) construction
  line L160 (-70.5279, -207.5692) -> (-70.0086, -207.234) construction
  line L161 (-70.0086, -207.234) -> (-69.5859, -206.9613) construction
  line L162 (-69.5859, -206.9613) -> (-69.5717, -206.2993) construction
  line L163 (-69.5717, -206.2993) -> (-69.913, -206.0081) construction
  line L164 (-69.913, -206.0081) -> (-69.9221, -205.8996) construction
  spline S12 degree 3 poles (-69.913, -206.0081) (-69.9221, -205.8996) (-69.9526, -205.7442) (-69.9564, -205.6719) knots 8.458233 8.458233 8.458233 8.458233 9 9 9 9
  line L165 (-69.9221, -205.8996) -> (-69.9526, -205.7442) construction
  line L166 (-69.9526, -205.7442) -> (-69.9564, -205.6719) construction
  line L167 (-69.9564, -205.6719) -> (-69.9688, -205.4394) construction
  spline S13 degree 3 poles (-69.9564, -205.6719) (-69.9688, -205.4394) (-69.9804, -205.2068) (-69.9922, -204.9742) knots 9 9 9 9 10 10 10 10
  line L168 (-69.9688, -205.4394) -> (-69.9804, -205.2068) construction
  line L169 (-69.9804, -205.2068) -> (-69.9922, -204.9742) construction
  line L170 (-65.21, -207.5244) -> (-64.6335, -206.4883) construction
  spline S14 degree 3 poles (-69.9958, -200.1973) (-70.0789, -200.257) (-70.116, -200.2834) (-70.1929, -200.3351) (-70.9193, -200.8239) (-71.9426, -201.315) (-71.7621, -202.3705) (-71.5629, -203.535) (-70.255, -203.6473) (-69.317, -203.8485) (-68.7434, -203.9715) (-68.1698, -204.0946) (-67.5962, -204.2176) (-67.2081, -204.3008) (-66.4341, -204.3449) (-66.1851, -204.6984) (-65.651, -205.4568) (-67.1637, -206.601) (-67.6138, -207.0402) (-68.5654, -207.9688) (-69.6689, -208.8594) (-70.4881, -209.9073) (-71.2068, -210.8265) (-71.435, -212.0475) (-70.3577, -212.7822) (-69.6264, -213.281) (-68.8425, -212.3276) (-69.211, -211.6355) (-69.348, -211.3783) (-68.7113, -210.8189) (-68.5641, -210.6697) (-68.0699, -210.1683) (-67.5704, -209.6721) (-67.0736, -209.1733) (-66.2478, -208.3442) (-65.21, -207.5244) (-64.6335, -206.4883) (-64.0778, -205.4895) (-64.0474, -204.1357) (-64.9252, -203.3045) (-65.7575, -202.5164) (-67.0963, -202.4289) (-68.1629, -202.2049) (-68.4721, -202.1399) (-68.7814, -202.075) (-69.0906, -202.01) (-69.1572, -201.996) (-69.2759, -201.9583) (-69.4064, -201.9194) knots 2.88117 2.88117 2.88117 2.88117 3 3 3 4 4 4 5 5 5 6 6 6 7 7 7 8 8 8 9 9 9 10 10 10 11 11 11 12 12 12 13 13 13 14 14 14 15 15 15 16 16 16 17 17 17 17.368094 17.368094 17.368094 17.368094
  line L171 (-69.9958, -200.1973) -> (-70.0789, -200.257) construction
  line L172 (-70.0789, -200.257) -> (-70.116, -200.2834) construction
  line L173 (-70.116, -200.2834) -> (-70.1929, -200.3351) construction
  line L174 (-70.1929, -200.3351) -> (-70.9193, -200.8239) construction
  line L175 (-70.9193, -200.8239) -> (-71.9426, -201.315) construction
  line L176 (-71.9426, -201.315) -> (-71.7621, -202.3705) construction
  line L177 (-71.7621, -202.3705) -> (-71.5629, -203.535) construction
  line L178 (-71.5629, -203.535) -> (-70.255, -203.6473) construction
  line L179 (-70.255, -203.6473) -> (-69.317, -203.8485) construction
  line L180 (-69.317, -203.8485) -> (-68.7434, -203.9715) construction
  line L181 (-68.7434, -203.9715) -> (-68.1698, -204.0946) construction
  line L182 (-68.1698, -204.0946) -> (-67.5962, -204.2176) construction
  line L183 (-67.5962, -204.2176) -> (-67.2081, -204.3008) construction
  line L184 (-67.2081, -204.3008) -> (-66.4341, -204.3449) construction
  line L185 (-66.4341, -204.3449) -> (-66.1851, -204.6984) construction
  line L186 (-66.1851, -204.6984) -> (-65.651, -205.4568) construction
  line L187 (-65.651, -205.4568) -> (-67.1637, -206.601) construction
  line L188 (-67.1637, -206.601) -> (-67.6138, -207.0402) construction
  line L189 (-67.6138, -207.0402) -> (-68.5654, -207.9688) construction
  line L190 (-68.5654, -207.9688) -> (-69.6689, -208.8594) construction
  line L191 (-69.6689, -208.8594) -> (-70.4881, -209.9073) construction
  line L192 (-70.4881, -209.9073) -> (-71.2068, -210.8265) construction
  line L193 (-71.2068, -210.8265) -> (-71.435, -212.0475) construction
  line L194 (-71.435, -212.0475) -> (-70.3577, -212.7822) construction
  line L195 (-70.3577, -212.7822) -> (-69.6264, -213.281) construction
  line L196 (-69.6264, -213.281) -> (-68.8425, -212.3276) construction
  line L197 (-68.8425, -212.3276) -> (-69.211, -211.6355) construction
  line L198 (-69.211, -211.6355) -> (-69.348, -211.3783) construction
  line L199 (-69.348, -211.3783) -> (-68.7113, -210.8189) construction
  line L200 (-68.7113, -210.8189) -> (-68.5641, -210.6697) construction
  line L201 (-68.5641, -210.6697) -> (-68.0699, -210.1683) construction
  line L202 (-68.0699, -210.1683) -> (-67.5704, -209.6721) construction
  line L203 (-67.5704, -209.6721) -> (-67.0736, -209.1733) construction
  line L204 (-67.0736, -209.1733) -> (-66.2478, -208.3442) construction
  line L205 (-66.2478, -208.3442) -> (-65.21, -207.5244) construction
  line L206 (-64.6335, -206.4883) -> (-64.0778, -205.4895) construction
  line L207 (-64.0778, -205.4895) -> (-64.0474, -204.1357) construction
  line L208 (-64.0474, -204.1357) -> (-64.9252, -203.3045) construction
  line L209 (-64.9252, -203.3045) -> (-65.7575, -202.5164) construction
  line L210 (-65.7575, -202.5164) -> (-67.0963, -202.4289) construction
  line L211 (-67.0963, -202.4289) -> (-68.1629, -202.2049) construction
  line L212 (-68.1629, -202.2049) -> (-68.4721, -202.1399) construction
  line L213 (-68.4721, -202.1399) -> (-68.7814, -202.075) construction
  line L214 (-68.7814, -202.075) -> (-69.0906, -202.01) construction
  line L215 (-69.0906, -202.01) -> (-69.1572, -201.996) construction
  line L216 (-69.1572, -201.996) -> (-69.2759, -201.9583) construction
  line L217 (-69.2759, -201.9583) -> (-69.4064, -201.9194) construction
  line L218 (-69.9922, -204.9742) -> (-70.0137, -204.5505) construction
  spline S15 degree 3 poles (-69.9922, -204.9742) (-70.0137, -204.5505) (-70.0308, -204.1271) (-70.0365, -203.7031) knots 10 10 10 10 10.82684 10.82684 10.82684 10.82684
  line L219 (-70.0137, -204.5505) -> (-70.0308, -204.1271) construction
  line L220 (-70.0308, -204.1271) -> (-70.0365, -203.7031) construction
  line L221 (-62.7613, -204.0034) -> (-62.8534, -205.0974) construction
  spline S16 degree 3 poles (-62.6293, -201.8117) (-62.6835, -202.9082) (-62.7613, -204.0034) (-62.8534, -205.0974) (-62.9738, -206.5259) (-63.1298, -207.9522) (-63.3323, -209.3714) (-63.5366, -210.8042) (-63.8561, -212.2768) (-63.8447, -213.7275) (-63.8371, -214.6872) (-62.6085, -214.7252) (-62.2826, -213.9389) (-61.4961, -212.0415) (-61.3373, -209.8217) (-61.0926, -207.7991) (-60.8465, -205.7642) (-60.6839, -203.7221) (-60.6094, -201.6738) (-60.5947, -201.2686) (-60.5808, -200.863) (-60.573, -200.4574) knots 5.14687 5.14687 5.14687 5.14687 6 6 6 7 7 7 8 8 8 9 9 9 10 10 10 11 11 11 11.773986 11.773986 11.773986 11.773986
  line L222 (-62.6293, -201.8117) -> (-62.6835, -202.9082) construction
  line L223 (-62.6835, -202.9082) -> (-62.7613, -204.0034) construction
  line L224 (-62.8534, -205.0974) -> (-62.9738, -206.5259) construction
  line L225 (-62.9738, -206.5259) -> (-63.1298, -207.9522) construction
  line L226 (-63.1298, -207.9522) -> (-63.3323, -209.3714) construction
  line L227 (-63.3323, -209.3714) -> (-63.5366, -210.8042) construction
  line L228 (-63.5366, -210.8042) -> (-63.8561, -212.2768) construction
  line L229 (-63.8561, -212.2768) -> (-63.8447, -213.7275) construction
  line L230 (-63.8447, -213.7275) -> (-63.8371, -214.6872) construction
  line L231 (-63.8371, -214.6872) -> (-62.6085, -214.7252) construction
  line L232 (-62.6085, -214.7252) -> (-62.2826, -213.9389) construction
  line L233 (-62.2826, -213.9389) -> (-61.4961, -212.0415) construction
  line L234 (-61.4961, -212.0415) -> (-61.3373, -209.8217) construction
  line L235 (-61.3373, -209.8217) -> (-61.0926, -207.7991) construction
  line L236 (-61.0926, -207.7991) -> (-60.8465, -205.7642) construction
  line L237 (-60.8465, -205.7642) -> (-60.6839, -203.7221) construction
  line L238 (-60.6839, -203.7221) -> (-60.6094, -201.6738) construction
  line L239 (-60.6094, -201.6738) -> (-60.5947, -201.2686) construction
  line L240 (-60.5947, -201.2686) -> (-60.5808, -200.863) construction
  line L241 (-60.5808, -200.863) -> (-60.573, -200.4574) construction
  line L242 (-69.2112, -201.78) -> (-69.0199, -201.6353) construction
  spline S17 degree 3 poles (-69.4064, -201.9194) (-69.2112, -201.78) (-69.0199, -201.6353) (-68.8331, -201.4851) (-68.0074, -200.8213) (-66.9016, -199.8854) (-66.5906, -198.831) (-65.8674, -196.379) (-69.0717, -195.9878) (-70.71, -196.1846) (-73.1638, -196.4794) (-75.594, -197.6595) (-77.1829, -199.5793) (-77.7742, -200.2938) (-76.8346, -201.286) (-76.1471, -200.6151) knots 21.261625 21.261625 21.261625 21.261625 22 22 22 23 23 23 24 24 24 25 25 25 26 26 26 26
  line L243 (-69.4064, -201.9194) -> (-69.2112, -201.78) construction
  line L244 (-69.0199, -201.6353) -> (-68.8331, -201.4851) construction
  line L245 (-68.8331, -201.4851) -> (-68.0074, -200.8213) construction
  line L246 (-68.0074, -200.8213) -> (-66.9016, -199.8854) construction
  line L247 (-66.9016, -199.8854) -> (-66.5906, -198.831) construction
  line L248 (-66.5906, -198.831) -> (-65.8674, -196.379) construction
  line L249 (-65.8674, -196.379) -> (-69.0717, -195.9878) construction
  line L250 (-69.0717, -195.9878) -> (-70.71, -196.1846) construction
  line L251 (-70.71, -196.1846) -> (-73.1638, -196.4794) construction
  line L252 (-73.1638, -196.4794) -> (-75.594, -197.6595) construction
  line L253 (-75.594, -197.6595) -> (-77.1829, -199.5793) construction
  line L254 (-77.1829, -199.5793) -> (-77.7742, -200.2938) construction
  line L255 (-77.7742, -200.2938) -> (-76.8346, -201.286) construction
  line L256 (-76.8346, -201.286) -> (-76.1471, -200.6151) construction
  line L257 (-68.6601, -197.5195) -> (-68.2505, -198.1283) construction
  spline S18 degree 3 poles (-76.1471, -200.6151) (-74.6694, -199.1729) (-72.8876, -198.1634) (-70.8255, -197.8634) (-70.2547, -197.7804) (-68.6601, -197.5195) (-68.2505, -198.1283) (-67.9248, -198.6124) (-69.3798, -199.7541) (-69.9958, -200.1973) knots 0 0 0 0 1 1 1 2 2 2 2.88117 2.88117 2.88117 2.88117
  line L258 (-76.1471, -200.6151) -> (-74.6694, -199.1729) construction
  line L259 (-74.6694, -199.1729) -> (-72.8876, -198.1634) construction
  line L260 (-72.8876, -198.1634) -> (-70.8255, -197.8634) construction
  line L261 (-70.8255, -197.8634) -> (-70.2547, -197.7804) construction
  line L262 (-70.2547, -197.7804) -> (-68.6601, -197.5195) construction
  line L263 (-68.2505, -198.1283) -> (-67.9248, -198.6124) construction
  line L264 (-67.9248, -198.6124) -> (-69.3798, -199.7541) construction
  line L265 (-69.3798, -199.7541) -> (-69.9958, -200.1973) construction
  line L266 (-62.7788, -200.0243) -> (-62.8676, -200.065) construction
  spline S19 degree 3 poles (-62.6111, -199.9275) (-62.6934, -199.9782) (-62.7788, -200.0243) (-62.8676, -200.065) (-63.5189, -200.3634) (-64.4227, -200.3174) (-64.9296, -199.7617) (-65.3787, -199.2694) (-65.3082, -198.5143) (-64.828, -198.0865) (-64.2177, -197.5428) (-65.0462, -196.4307) (-65.7156, -196.9363) knots 16.74527 16.74527 16.74527 16.74527 17 17 17 18 18 18 19 19 19 20 20 20 20
  line L267 (-62.6111, -199.9275) -> (-62.6934, -199.9782) construction
  line L268 (-62.6934, -199.9782) -> (-62.7788, -200.0243) construction
  line L269 (-62.8676, -200.065) -> (-63.5189, -200.3634) construction
  line L270 (-63.5189, -200.3634) -> (-64.4227, -200.3174) construction
  line L271 (-64.4227, -200.3174) -> (-64.9296, -199.7617) construction
  line L272 (-64.9296, -199.7617) -> (-65.3787, -199.2694) construction
  line L273 (-65.3787, -199.2694) -> (-65.3082, -198.5143) construction
  line L274 (-65.3082, -198.5143) -> (-64.828, -198.0865) construction
  line L275 (-64.828, -198.0865) -> (-64.2177, -197.5428) construction
  line L276 (-64.2177, -197.5428) -> (-65.0462, -196.4307) construction
  line L277 (-65.0462, -196.4307) -> (-65.7156, -196.9363) construction
  line L278 (-65.647, -201.3697) -> (-64.7256, -202.0352) construction
  spline S20 degree 3 poles (-65.7156, -196.9363) (-67.2086, -198.064) (-67.1719, -200.2683) (-65.647, -201.3697) (-64.7256, -202.0352) (-63.6312, -202.1196) (-62.6293, -201.8117) knots 0 0 0 0 1 1 1 1.551759 1.551759 1.551759 1.551759
  line L279 (-65.7156, -196.9363) -> (-67.2086, -198.064) construction
  line L280 (-67.2086, -198.064) -> (-67.1719, -200.2683) construction
  line L281 (-67.1719, -200.2683) -> (-65.647, -201.3697) construction
  line L282 (-64.7256, -202.0352) -> (-63.6312, -202.1196) construction
  line L283 (-63.6312, -202.1196) -> (-62.6293, -201.8117) construction
  line L284 (-60.573, -200.4574) -> (-60.5526, -200.4338) construction
  spline S21 degree 3 poles (-60.573, -200.4574) (-60.5526, -200.4338) (-60.5326, -200.41) (-60.5128, -200.386) (-59.9126, -199.658) (-59.306, -198.6179) (-59.9276, -197.7182) (-60.5269, -196.8506) (-61.7546, -196.9592) (-62.2545, -197.8573) (-62.5725, -198.4287) (-62.6155, -199.1887) (-62.6111, -199.9275) knots 1.983848 1.983848 1.983848 1.983848 2 2 2 3 3 3 4 4 4 4.613609 4.613609 4.613609 4.613609
  line L285 (-60.5526, -200.4338) -> (-60.5326, -200.41) construction
  line L286 (-60.5326, -200.41) -> (-60.5128, -200.386) construction
  line L287 (-60.5128, -200.386) -> (-59.9126, -199.658) construction
  line L288 (-59.9126, -199.658) -> (-59.306, -198.6179) construction
  line L289 (-59.306, -198.6179) -> (-59.9276, -197.7182) construction
  line L290 (-59.9276, -197.7182) -> (-60.5269, -196.8506) construction
  line L291 (-60.5269, -196.8506) -> (-61.7546, -196.9592) construction
  line L292 (-61.7546, -196.9592) -> (-62.2545, -197.8573) construction
  line L293 (-62.2545, -197.8573) -> (-62.5725, -198.4287) construction
  line L294 (-62.5725, -198.4287) -> (-62.6155, -199.1887) construction
  line L295 (-62.6155, -199.1887) -> (-62.6111, -199.9275) construction
  circle A1 centre (-61.0467, -198.6179) radius 0.6286
  line L296 (-77.3718, -179.3764) -> (-76.5866, -179.6814) construction
  spline S22 degree 3 poles (-75.895, -170.0979) (-76.1064, -169.2219) (-77.4372, -169.018) (-77.8095, -170.0542) (-78.4611, -171.8676) (-78.2971, -174.2243) (-78.203, -176.1264) (-78.1641, -176.9137) (-78.2111, -178.0238) (-77.7818, -178.7157) (-77.3718, -179.3764) (-76.5866, -179.6814) (-75.9115, -179.2457) (-75.362, -178.8911) (-75.3436, -178.0305) (-75.7872, -177.652) knots 1.141449 1.141449 1.141449 1.141449 2 2 2 3 3 3 4 4 4 5 5 5 5.747549 5.747549 5.747549 5.747549
  line L297 (-75.895, -170.0979) -> (-76.1064, -169.2219) construction
  line L298 (-76.1064, -169.2219) -> (-77.4372, -169.018) construction
  line L299 (-77.4372, -169.018) -> (-77.8095, -170.0542) construction
  line L300 (-77.8095, -170.0542) -> (-78.4611, -171.8676) construction
  line L301 (-78.4611, -171.8676) -> (-78.2971, -174.2243) construction
  line L302 (-78.2971, -174.2243) -> (-78.203, -176.1264) construction
  line L303 (-78.203, -176.1264) -> (-78.1641, -176.9137) construction
  line L304 (-78.1641, -176.9137) -> (-78.2111, -178.0238) construction
  line L305 (-78.2111, -178.0238) -> (-77.7818, -178.7157) construction
  line L306 (-77.7818, -178.7157) -> (-77.3718, -179.3764) construction
  line L307 (-76.5866, -179.6814) -> (-75.9115, -179.2457) construction
  line L308 (-75.9115, -179.2457) -> (-75.362, -178.8911) construction
  line L309 (-75.362, -178.8911) -> (-75.3436, -178.0305) construction
  line L310 (-75.3436, -178.0305) -> (-75.7872, -177.652) construction
  line L311 (-74.8747, -184.9677) -> (-75.0528, -184.6332) construction